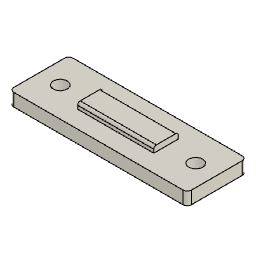
LED PCB Spacer (Autodesk Fusion 360 design; units mm, degrees)
Autodesk Fusion 360 part; units mm, degrees
sketch "Sketch1" plane through (0, 0, 0) normal (0, 0, 1) x (1, 0, 0)
  line L0 (21, 7) -> (-21, 7)
  line L1 (-21, 7) -> (-21, -7)
  line L2 (-21, -7) -> (21, -7)
  line L3 (21, -7) -> (21, 7)
  line L4 (21, 7) -> (-21, -7) construction
  line L5 (-21, 7) -> (21, -7) construction
  line L6 (-16, 0) -> (16, 0) construction
  circle A0 centre (-16, 0) radius 2.35
  circle A1 centre (16, 0) radius 2.35
  dimension "d1" = 14
  dimension "d2" = 42
  dimension "d3" = 32
  dimension "d4" = 4.7
  constraint horizontal L0
  constraint perpendicular L0 L1
  constraint parallel L0 L2
  constraint parallel L1 L3
  constraint coincident L4 origin
  constraint coincident L5 origin
  constraint parallel L2 L6
  constraint midpoint origin L6
  constraint coincident L6.start A0.centre
  constraint coincident L6.end A1.centre
  constraint equal A0 A1
  measures "d1" distance of L0.start L2.end
  measures "d2" distance of L0.start L0.end
  measures "d3" distance of L6.start L6.end
  measures "d4" diameter of A1
extrude "Extrude1" add sketch "Sketch1" along normal blind 3 contours L0 L1 L2 L3 | A0 | A1
sketch "Sketch2" plane through (0, 0, 3) normal (0, 0, 1) x (-1, 0, 0)
  line L0 (-21, 7) -> (-21, -7)
  line L1 (-21, -7) -> (21, -7)
  line L2 (21, -7) -> (21, 7)
  line L3 (21, 7) -> (-21, 7)
  line L4 (16, 0) -> (-16, 0) construction
  dimension "d7" = 32
  constraint parallel L3 L4
  constraint midpoint origin L4
  measures "d7" distance of L4.start L4.end
hole "Hole1" at (-16, 0, 3) at (16, 0, 3) direction (0, 0, -1) diameter 3.3 depth 5 tip angle 180
sketch "Sketch3" plane through (0, 0, 0) normal (0, 0, -1) x (-1, 0, 0)
  circle A0 centre (16, 0) radius 1.65
  circle A1 centre (-16, 0) radius 1.65
  line L0 (-21, 6) -> (-21, -6)
  line L1 (-21, -6) -> (21, -6)
  line L2 (21, -6) -> (21, 6)
  line L3 (21, 6) -> (-21, 6)
  circle A2 centre (16, 0) radius 1.65
  circle A3 centre (-16, 0) radius 1.65
  line L4 (-21, 7) -> (-21, -7)
  line L5 (-21, -7) -> (21, -7)
  line L6 (21, -7) -> (21, 7)
  line L7 (21, 7) -> (-21, 7)
  line L8 (-12, -2) -> (12, -2)
  line L9 (12, -2) -> (12, 2)
  line L10 (12, 2) -> (-12, 2)
  line L11 (-12, 2) -> (-12, -2)
  line L12 (-12, -2) -> (12, 2) construction
  line L13 (12, -2) -> (-12, 2) construction
  dimension "d11" = 4
  dimension "d12" = 24
  constraint horizontal L8
  constraint perpendicular L8 L9
  constraint parallel L8 L10
  constraint parallel L9 L11
  constraint coincident L12 origin
  constraint coincident L13 origin
  measures "d11" distance of L8.start L10.end
  measures "d12" distance of L8.start L8.end
extrude "Extrude2" cut sketch "Sketch3" against normal blind 2 contours L8 L9 L10 L11
sketch "Sketch4" plane through (0, 0, 3) normal (0, 0, 1) x (-1, 0, 0)
  circle A0 centre (16, 0) radius 1.65
  circle A1 centre (-16, 0) radius 1.65
  line L0 (-21, 7) -> (-21, -7)
  line L1 (-21, -7) -> (21, -7)
  line L2 (21, -7) -> (21, 7)
  line L3 (21, 7) -> (-21, 7)
  line L4 (-9, -2.9) -> (9, -2.9)
  line L5 (9, -2.9) -> (9, 2.9)
  line L6 (9, 2.9) -> (-9, 2.9)
  line L7 (-9, 2.9) -> (-9, -2.9)
  line L8 (-9, -2.9) -> (9, 2.9) construction
  line L9 (9, -2.9) -> (-9, 2.9) construction
  dimension "d15" = 5.8
  dimension "d16" = 18
  constraint horizontal L4
  constraint perpendicular L4 L5
  constraint parallel L4 L6
  constraint parallel L5 L7
  constraint coincident L8 origin
  constraint coincident L9 origin
  measures "d15" distance of L4.start L6.end
  measures "d16" distance of L4.start L4.end
extrude "Extrude3" add sketch "Sketch4" along normal blind 1.4 contours L4 L5 L6 L7
fillet "Fillet1" radius 0.6 2 edges at (0, -2.9, 4.4) (0, 2.9, 4.4)
fillet "Fillet2" radius 1 4 edges at (-21, 7, 1.5) (21, 7, 1.5) (21, -7, 1.5) (-21, -7, 1.5)
